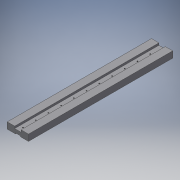
# Autodesk Inventor part: Zcolumn
Saved by Autodesk Inventor 2019 (Build 230136000, 136)
## iProperties
Created: 2018-10-03
Part Number: Zcolumn
Material: Generic
Document SubType Name: Modeling
Designer: LillaHunden
Density: 1 g/cm^3
Appearance: Default
Author: LillaHunden
Autodesk Inventor part; units mm, degrees
ref_plane "YZ Plane" through (0, 0, 0) normal (1, 0, 0) x (0, 1, 0)
ref_plane "XZ Plane" through (0, 0, 0) normal (0, 1, 0) x (-1, 0, 0)
ref_plane "XY Plane" through (0, 0, 0) normal (0, 0, 1) x (1, 0, 0)
sketch "Sketch1" plane through (0, 0, 0) normal (0, 0, 1) x (1, 0, 0)
  line L0 (-83.9793, 28.2703) -> (-133.9793, 28.2703)
  line L1 (-133.9793, 28.2703) -> (-133.9793, 43.2703)
  line L2 (-133.9793, 43.2703) -> (-83.9793, 43.2703)
  line L3 (-83.9793, 43.2703) -> (-83.9793, 28.2703)
  point P0 (0, 0)
  dimension "d0" = 50
  dimension "d1" = 15
  constraints: 8 end point, 2 parallel, 1 horizontal, 1 perpendicular
  measures "d0" distance of L1.end L2.end
  measures "d1" distance of L0.end L1.end
extrude "Extrusion1" add sketch "Sketch1" along normal blind 340
sketch "Sketch2" plane through (-133.9793, 43.2703, 0) normal (0, 1, 0) x (1, 0, 0)
  line L0 (50, 0) -> (0, 0) projected
  line L1 (32.55, -340) -> (17.45, -340)
  line L2 (17.45, -340) -> (17.45, 0)
  line L3 (17.45, 0) -> (32.55, 0)
  line L4 (32.55, 0) -> (32.55, -340)
  line L5 (50, -340) -> (0, -340) projected
  point P0 (133.9793, 0)
  point P1 (25, -340)
  dimension "d4" = 15.1
  constraints: 8 end point, 2 midpoint, 2 parallel, 1 horizontal, 1 perpendicular, 1 point on line
  measures "d4" distance between parallel lines of L4 L2
extrude "Extrusion2" cut sketch "Sketch2" against normal blind 5
sketch "Sketch3" plane through (-133.9793, 28.2703, 0) normal (0, -1, 0) x (1, 0, 0)
  line L0 (17.45, 340) -> (0, 340) projected
  line L1 (17.45, 0) -> (32.55, 0) projected
  line L2 (19, 340) -> (31, 340)
  line L3 (31, 340) -> (31, 0)
  line L4 (31, 0) -> (19, 0)
  line L5 (19, 0) -> (19, 340)
  line L6 (0, 340) -> (50, 340) projected
  point P0 (133.9793, 0)
  point P1 (25, 340)
  dimension "d7" = 12
  constraints: 8 end point, 2 midpoint, 2 parallel, 2 point on line, 1 horizontal, 1 perpendicular
  measures "d7" distance of L3.end L4.end
extrude "Extrusion3" cut sketch "Sketch3" against normal blind 2
body "Solid1"
